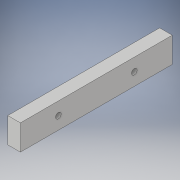
# Autodesk Inventor part: RestForCuts
Saved by Autodesk Inventor 2019 (Build 230136000, 136)
## iProperties
Created: 2018-07-14
Part Number: RestForCuts
Material: Generic
Document SubType Name: Modeling
Designer: steele
Density: 1 g/cm^3
Appearance: Default
Author: steele
Autodesk Inventor part; units mm, degrees
ref_plane "YZ Plane" through (0, 0, 0) normal (1, 0, 0) x (0, 1, 0)
ref_plane "XZ Plane" through (0, 0, 0) normal (0, 1, 0) x (-1, 0, 0)
ref_plane "XY Plane" through (0, 0, 0) normal (0, 0, 1) x (1, 0, 0)
sketch "Sketch2" plane through (0, 0, 0) normal (0, 0, 1) x (1, 0, 0)
  line L0 (0, 0) -> (12.7, 0)
  line L1 (12.7, 0) -> (12.7, 50.8)
  line L2 (12.7, 50.8) -> (0, 50.8)
  line L3 (0, 0) -> (0, 50.8) construction
  line L4 (0, 0) -> (-12.7, 0)
  line L5 (-12.7, 0) -> (-12.7, 50.8)
  line L6 (-12.7, 50.8) -> (0, 50.8)
  dimension "d0" = 12.7
  dimension "d1" = 50.8
  constraints: 14 end point, 2 perpendicular, 2 symmetric about line, 1 horizontal, 1 vertical
  measures "d0" distance of L1.end L2.end
  measures "d1" distance of L0.end L1.end
extrude "Extrusion1" add sketch "Sketch2" along normal mid plane 304.8
sketch "Sketch3" plane through (12.7, 0, 152.4) normal (1, 0, 0) x (0, 0, -1)
  line L0 (0, 0) -> (0, 50.8) construction
  line L1 (0, 25.4) -> (304.8, 25.4) construction
  line L2 (304.8, 50.8) -> (304.8, 0) construction
  point P0 (152.4, 0)
  point P1 (76.2, 25.4)
  point P2 (228.6, 25.4)
  point P3 (184.7909, 73.7254)
  dimension "d4" = 76.2
  dimension "d5" = 76.2
  constraints: 2 end point, 2 midpoint, 2 point on line
  measures "d4" distance from line of L0 point (76.2, 25.4)
  measures "d5" distance from line of point (228.6, 25.4) L2
hole "Hole1" at (12.7, 25.4, 76.2) at (12.7, 25.4, -76.2) at (12.7, 73.7254, -32.3909) direction (-1, 0, 0) diameter 6.7564 end through all counterbore diameter 11.1252 counterbore depth 34.29 clearance for "Socket Head Cap Screw" size "1/4" standard "Ansi Unified Screw Threads"
body "Solid1"
